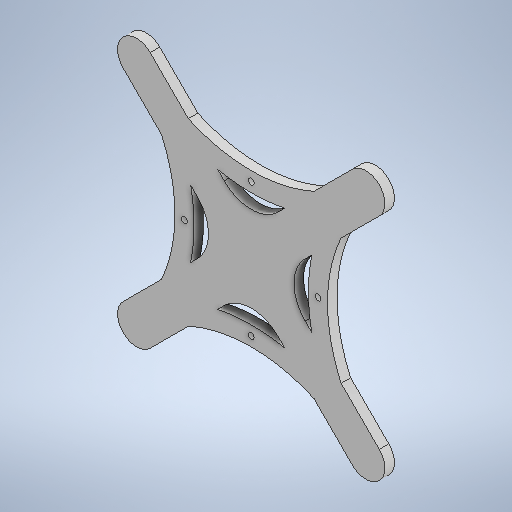
# Autodesk Inventor part: Base
Saved by Autodesk Inventor 2025.1 (Build 291241020, 241B)
## iProperties
Created: 2024-09-22
Part Number: Base
Material: 일반
Document SubType Name: Modeling
Designer: daare
Density: 1 g/cm^3
Appearance: 기본값
Author: daare
Autodesk Inventor part; units mm, degrees
ref_plane "YZ Plane" through (0, 0, 0) normal (1, 0, 0) x (0, 1, 0)
ref_plane "XZ Plane" through (0, 0, 0) normal (0, 1, 0) x (-1, 0, 0)
ref_plane "XY Plane" through (0, 0, 0) normal (0, 0, 1) x (1, 0, 0)
sketch "스케치1" plane through (0, 0, 0) normal (0, 0, 1) x (1, 0, 0)
  arc A0 (-52.9289, 67.0711) -> (-67.0711, 52.9289) centre (-60, 60) ccw
  line L0 (-67.0711, 52.9289) -> (-28.2843, 14.1421)
  line L1 (-52.9289, 67.0711) -> (-14.1421, 28.2843)
  line L2 (-60, 60) -> (0, 0)
  arc A1 (-22.4264, 0) -> (-28.2843, 14.1421) centre (-42.4264, 0) ccw
  line L3 (-152.003, 0) -> (72.0182, 0) projected
  arc A2 (-14.1421, 28.2843) -> (0, 22.4264) centre (0, 42.4264) ccw
  line L4 (0, -72.0182) -> (0, 152.003) projected
  arc A3 (-47.1079, -32.9658) -> (-47.1079, 32.9658) centre (-120, 0) ccw
  arc A4 (-39.0886, -39.4124) -> (-31.7366, 17.5944) centre (-120, 0) ccw
  line L5 (-40, 0) -> (-30, 0)
  arc A5 (-32.9658, 47.1079) -> (32.9658, 47.1079) centre (0, 120) ccw
  arc A6 (-17.5944, 31.7366) -> (39.4124, 39.0886) centre (0, 120) ccw
  circle A7 centre (-35, 0) radius 1.5
  circle A8 centre (0, 35) radius 1.5
  point P0 (-17.5944, 31.7366)
  point P1 (0, 30)
  point P2 (0, 40)
  point P3 (-32.9658, 47.1079)
  point P4 (-40, 0)
  point P5 (-36.5, 0)
  point P6 (-33.5, 0)
  point P7 (0, 33.5)
  point P8 (0, 36.5)
  dimension "d0" = 60
  dimension "d1" = 60
  dimension "d2" = 20
  dimension "d3" = 20
  dimension "d29" = 10
  dimension "d30" = 35
  dimension "d31" = 80
  dimension "d32" = 3
  constraints: 16 point on circle, 9 centre point, 9 symmetric about line, 8 end point, 4 point on line, 3 tangent, 2 horizontal alignment, 2 parallel, 1 coincident, 1 midpoint, 1 vertical alignment, 4 other
  measures "d0" horizontal distance of L2.end L2.start
  measures "d1" horizontal distance of L2.end L2.start
  measures "d2" diameter of A0
  measures "d3" radius of A1
  measures "d29" radial gap between concentric circles of A3 A4
  measures "d30" distance of L2.end point (-35, 0)
  measures "d31" radius of A3
  measures "d32" diameter of A7
extrude "돌출1" add sketch "스케치1" along normal blind 5 contours L1 A2 L4 L3 A1 L0 A0 | A5 L4 A8 A6 L1 | L0 A4 L3 A7 A3
pattern_circular "원형 패턴1" count 4 over 360 about axis through (0, 0, -10) along (0, 0, 1) of "돌출1"
